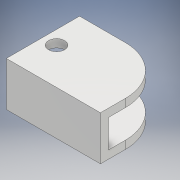
# Autodesk Inventor part: Finger2
Saved by Autodesk Inventor 2018 (Build 220112000, 112)
## iProperties
Created: 2018-02-19
Part Number: Finger2
Material: Plastique ABS
Document SubType Name: Modeling
Designer: Thomas
Density: 1.06 g/cm^3
Appearance: Lisse - Blanc
Author: Thomas
Autodesk Inventor part; units mm, degrees
ref_plane "YZ Plane" through (0, 0, 0) normal (1, 0, 0) x (0, 1, 0)
ref_plane "XZ Plane" through (0, 0, 0) normal (0, 1, 0) x (-1, 0, 0)
ref_plane "XY Plane" through (0, 0, 0) normal (0, 0, 1) x (1, 0, 0)
sketch "Esquisse1" plane through (0, 0, 0) normal (0, 0, 1) x (1, 0, 0)
  line L0 (0, 0) -> (23.4, 0)
  line L1 (23.4, 0) -> (23.4, 6.2)
  line L2 (11.4, 18.2) -> (0, 18.2)
  line L3 (0, 18.2) -> (0, 0)
  arc A0 (23.4, 6.2) -> (11.4, 18.2) centre (11.4, 6.2) ccw
  dimension "d0" = 18.2
  dimension "d1" = 23.4
  dimension "d2" = 12
  constraints: 8 end point, 2 parallel, 2 point on circle, 2 tangent, 1 centre point, 1 horizontal, 1 perpendicular
  measures "d0" distance of L2.end L0.start
  measures "d1" distance of L0.start L0.end
  measures "d2" radius of A0
extrude "Extrusion1" add sketch "Esquisse1" along normal blind 2
sketch "Esquisse2" plane through (0, 0, 0) normal (0, -1, 0) x (1, 0, 0)
  line L0 (0, 2) -> (23.4, 2) projected
  line L1 (0, 2) -> (23.4, 2)
  line L2 (23.4, 2) -> (23.4, 11)
  line L3 (23.4, 11) -> (0, 11)
  line L4 (0, 11) -> (0, 2)
  point P0 (0, 0)
  dimension "d5" = 9
  constraints: 8 end point, 2 parallel, 1 horizontal, 1 perpendicular
  measures "d5" distance of L3.end L0.start
extrude "Extrusion2" add sketch "Esquisse2" against normal blind 2
sketch "Esquisse3" plane through (0, 0, 11) normal (0, 0, 1) x (1, 0, 0)
  line L0 (0, 2) -> (23.4, 2) projected
  line L1 (23.4, 2) -> (0, 2)
  line L2 (0, 2) -> (0, 18.2)
  line L3 (0, 18.2) -> (11.4, 18.2)
  line L4 (23.4, 6.2) -> (23.4, 2)
  arc A0 (23.4, 6.2) -> (11.4, 18.2) centre (11.4, 6.2) ccw
  point P0 (0, 0)
  dimension "d8" = 16.2
  dimension "d9" = 12
  constraints: 8 end point, 2 parallel, 2 point on circle, 2 tangent, 1 centre point, 1 horizontal, 1 perpendicular
  measures "d8" distance of L1.end L2.end
  measures "d9" radius of A0
extrude "Extrusion3" add sketch "Esquisse3" against normal blind 2
sketch "Esquisse4" plane through (0, 0, 11) normal (0, 0, 1) x (1, 0, 0)
  circle A0 centre (3.39, 9.1) radius 2
  line L0 (23.4, 0) -> (0, 0) projected
  line L1 (23.4, 0) -> (23.4, 6.2) projected
  line L2 (0, 0) -> (0, 18.2) projected
  dimension "d12" = 9.1
  dimension "d14" = 4
  dimension "d19" = 3.39
  constraints: 1 centre point
  measures "d12" distance from line of L0 A0.centre
  measures "d14" diameter of A0
  measures "d19" distance from line of L2 A0.centre
extrude "Extrusion4" cut sketch "Esquisse4" against normal blind 2
sketch "Esquisse5" plane through (0, 0, 0) normal (0, 0, -1) x (-1, 0, 0)
  circle A0 centre (-3.39, 9.1) radius 2 projected
  circle A1 centre (-3.39, 9.1) radius 2
  point P0 (0, 0)
  constraints: 1 centre point, 1 coincident
extrude "Extrusion5" cut sketch "Esquisse5" against normal blind 2
